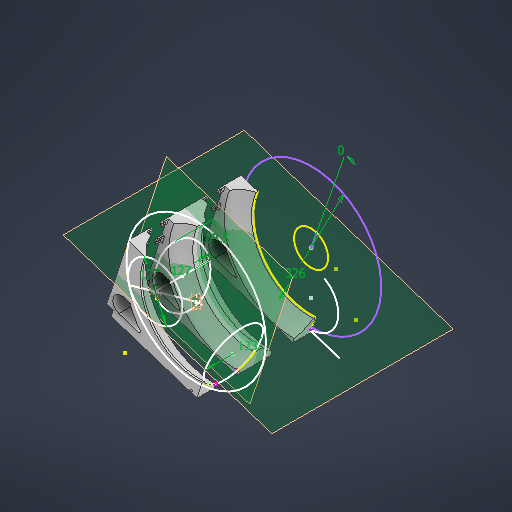
# Autodesk Inventor part: загиб 20-25
Saved by Autodesk Inventor 2025 (Build 290162000, 162)
## iProperties
Created: 2025-10-03
Part Number: загиб 20-25
Material: Типовые
Document SubType Name: Modeling
Designer: Phantom
Density: 1 g/cm^3
Appearance: По умолчанию
Author: Phantom
Autodesk Inventor part; units mm, degrees
ref_plane "YZ Plane" through (0, 0, 0) normal (1, 0, 0) x (0, 1, 0)
ref_plane "XZ Plane" through (0, 0, 0) normal (0, 1, 0) x (-1, 0, 0)
ref_plane "XY Plane" through (0, 0, 0) normal (0, 0, 1) x (1, 0, 0)
sketch "Эскиз1" plane through (0, 0, 0) normal (0, 0, 1) x (1, 0, 0)
  line L0 (14.5513, 220.3235) -> (16.6686, 220.3036)
  line L1 (220, 0) -> (230, 0) construction
  line L2 (0, 0) -> (170, 0)
  line L3 (170, 0) -> (170, 2)
  arc A0 (14.5513, 220.3235) -> (170, 0) centre (170, 165) ccw
  arc A1 (16.6686, 220.3036) -> (170, 2) centre (170, 165) ccw
  line L4 (170, 1) -> (170, 0)
  dimension "d12" = 330
  dimension "d13" = 2
  constraints: 10 end point, 4 point on circle, 2 centre point, 2 horizontal, 1 midpoint, 1 vertical
  measures "d12" diameter of A0
  measures "d13" radial gap between concentric circles of A0 A1
extrude "Выдавливание1" add sketch "Эскиз1" along normal blind 385
sketch "Эскиз2" plane through (0, 0, 0) normal (0, 0, -1) x (-1, 0, 0)
  line L0 (-16.6686, 220.3036) -> (-14.5513, 220.3235) projected
  arc A0 (-170, 2) -> (-16.6686, 220.3036) centre (-170, 165) ccw projected
  line L1 (-170, 0) -> (-170, 2) projected
  arc A1 (-170, 0) -> (-14.5513, 220.3235) centre (-170, 165) ccw projected
  point P0 (0, 0)
extrude "Выдавливание2" cut sketch "Эскиз2" against normal blind 121
chamfer "Фаска1" distance 2 angle 45 1 edges at (170, 2, 253)
chamfer "Фаска2" distance 2.8 angle 45 1 edges at (168.0001, 2.0123, 253)
sketch "Эскиз4" plane through (0, 0, 385) normal (0, 0, 1) x (1, 0, 0)
  line L0 (165.2006, 2.0707) -> (169.9739, 0.0263) projected
  arc A0 (16.6686, 220.3036) -> (165.2006, 2.0707) centre (170, 165) ccw projected
  line L1 (16.6686, 220.3036) -> (14.5513, 220.3235) projected
  arc A1 (14.5513, 220.3235) -> (170, 0) centre (170, 165) ccw projected
  line L2 (169.9739, 0.0263) -> (170, 0) projected
  arc A2 (8.48, 230.7703) -> (172.1929, 23.6823) centre (165.364, 186.5392) ccw projected
  arc A3 (6.3666, 230.6392) -> (177.1276, 21.959) centre (165.364, 186.5392) ccw projected
  line L3 (8.48, 230.7703) -> (6.3666, 230.6392) projected
  point P0 (0, 0)
  point P1 (6.736, 141.1283)
  point P2 (5.2437, 156.0352)
extrude "Выдавливание3" add sketch "Эскиз4" against normal up to surface (264 mm away) contours A3 L3 A2 A1
sketch "Эскиз5" plane through (0, 0, 385) normal (0, 0, 1) x (1, 0, 0)
  point P0 (0, 0)
sketch "Эскиз6" plane through (0, 0, 385) normal (0, 0, 1) x (1, 0, 0)
  arc A0 (8.48, 230.7703) -> (172.1929, 23.6823) centre (165.364, 186.5392) ccw projected
  arc A1 (4.2174, 151.0884) -> (177.1276, 21.959) centre (165.364, 186.5392) ccw projected
  arc A2 (6.3666, 230.6392) -> (6.736, 141.1283) centre (165.364, 186.5392) ccw projected
  line L0 (8.48, 230.7703) -> (6.3666, 230.6392) projected
  line L1 (165.2006, 2.0707) -> (169.9739, 0.0263) projected
  arc A3 (16.6686, 220.3036) -> (165.2006, 2.0707) centre (170, 165) ccw projected
  line L2 (16.6686, 220.3036) -> (14.5513, 220.3235) projected
  arc A4 (14.5513, 220.3235) -> (5.2437, 156.0352) centre (170, 165) ccw projected
  arc A5 (8.48, 230.7703) -> (5.2437, 156.0352) centre (165.364, 186.5392) ccw projected
  line L3 (8.48, 230.7703) -> (6.3666, 230.6392) projected
  arc A6 (6.3666, 230.6392) -> (6.736, 141.1283) centre (165.364, 186.5392) ccw projected
  arc A7 (6.736, 141.1283) -> (170, 0) centre (170, 165) ccw projected
  line L4 (169.9739, 0.0263) -> (170, 0) projected
  point P0 (0, 0)
  point P1 (5.2437, 156.0352)
  point P2 (8.6956, 141.5501)
extrude "Выдавливание4" cut sketch "Эскиз6" against normal through all contours A4 L2 A3 A0
sketch "Эскиз7" plane through (0, 0, 385) normal (0, 0, 1) x (1, 0, 0)
  arc A0 (8.48, 230.7703) -> (8.6956, 141.5501) centre (165.364, 186.5392) ccw projected
  line L0 (8.48, 230.7703) -> (6.3666, 230.6392) projected
  arc A1 (6.3666, 230.6392) -> (6.736, 141.1283) centre (165.364, 186.5392) ccw projected
  arc A2 (6.736, 141.1283) -> (170, 0) centre (170, 165) ccw projected
  line L1 (169.9739, 0.0263) -> (170, 0) projected
  line L2 (165.2006, 2.0707) -> (169.9739, 0.0263) projected
  arc A3 (8.6956, 141.5501) -> (165.2006, 2.0707) centre (170, 165) ccw projected
  line L3 (7.9507, 133.9351) -> (-40.0993, 149.5316)
  line L4 (-49.858, 62.7801) -> (67.4599, 424.2168) projected
  line L5 (-49.858, 62.7801) -> (127.0544, 5.6869)
  line L6 (-49.858, 62.7801) -> (-48.0056, 68.487)
  line L7 (-48.0056, 68.487) -> (101.3216, 20.2961)
  line L8 (86.2538, 25.1587) -> (84.4111, 19.4487)
  line L9 (-13.7205, 69.3639) -> (64.1078, 44.2472)
  line L10 (-13.7205, 69.3639) -> (-53.2073, 82.1071)
  line L11 (6.3666, 230.6392) -> (-61.8212, 20.5641)
  line L12 (0.3654, 112.7603) -> (33.0364, 102.1557)
  line L13 (0.3654, 112.7603) -> (-39.1966, 125.6017)
  point P0 (0, 0)
  point P1 (-42.9225, 78.788)
  point P2 (-48.2834, 62.2719)
  point P3 (85.6236, 23.2057)
  point P4 (54.2251, 47.4365)
  point P5 (-21.8795, 143.6177)
  point P6 (-28.8205, 122.2337)
  point P7 (15.1754, 107.9532)
  dimension "d24" = 6
  constraints: 20 end point, 4 parallel, 3 point on circle, 3 point on line, 2 perpendicular, 1 collinear, 2 other
  measures "d24" distance of L4.start L6.end
extrude "Выдавливание5" add sketch "Эскиз7" against normal up to surface (264 mm away) contours A1 A2 L3 L11 | L3 A2 L12 L13 L11 | A2 L7 L11 L10 L9 | A2 L8 L5 L11 L7
sketch "Эскиз8" plane through (0, 0, 385) normal (0, 0, 1) x (1, 0, 0)
  arc A0 (-12.5279, 69.512) -> (1.2437, 111.9401) centre (-8.4636, 91.6419) ccw projected
  arc A1 (15.1754, 107.9532) -> (54.2251, 47.4365) centre (170, 165) ccw projected
  arc A2 (9.1771, 109.9002) -> (50.7168, 43.874) centre (170, 165) ccw
  line L0 (-28.8205, 122.2337) -> (15.1754, 107.9532) projected
  line L1 (54.2251, 47.4365) -> (-42.9225, 78.788) projected
  point P0 (0, 0)
  point P1 (44.1807, 50.678)
  dimension "d27" = 5
  constraints: 2 point on circle, 1 centre point, 1 point on line
  measures "d27" radial gap between concentric circles of A1 A2
extrude "Выдавливание6" add sketch "Эскиз8" against normal up to surface (264 mm away)
sketch "Эскиз9" plane through (0, 0, 385) normal (0, 0, 1) x (1, 0, 0)
  arc A0 (8.48, 230.7703) -> (8.6956, 141.5501) centre (165.364, 186.5392) ccw projected
  line L0 (8.48, 230.7703) -> (6.3666, 230.6392) projected
  line L1 (6.3666, 230.6392) -> (-28.8205, 122.2337) projected
  line L2 (-28.8205, 122.2337) -> (9.1771, 109.9002) projected
  arc A1 (9.1771, 109.9002) -> (44.1807, 50.678) centre (170, 165) ccw projected
  line L3 (44.1807, 50.678) -> (-42.9225, 78.788) projected
  line L4 (-42.9225, 78.788) -> (-48.2834, 62.2719) projected
  line L5 (-48.2834, 62.2719) -> (84.4111, 19.4487) projected
  line L6 (84.4111, 19.4487) -> (85.6236, 23.2057) projected
  arc A2 (85.6236, 23.2057) -> (170, 0) centre (170, 165) ccw projected
  line L7 (169.9739, 0.0263) -> (170, 0) projected
  line L8 (165.2006, 2.0707) -> (169.9739, 0.0263) projected
  arc A3 (8.6956, 141.5501) -> (165.2006, 2.0707) centre (170, 165) ccw projected
  line L9 (85.6236, 23.2057) -> (90.4504, 38.1623)
  line L10 (84.4111, 19.4487) -> (85.6236, 23.2057) projected
  point P0 (0, 0)
  point P1 (86.2538, 25.1587)
  constraints: 2 end point, 1 collinear
extrude "Выдавливание7" cut sketch "Эскиз9" against normal through all contours A3 L8 L7 A2 L9
sketch "Эскиз10" plane through (0, 0, 385) normal (0, 0, 1) x (1, 0, 0)
  line L0 (8.48, 230.7703) -> (6.3666, 230.6392) projected
  line L1 (-48.2834, 62.2719) -> (6.3666, 230.6392)
  line L2 (-48.2834, 62.2719) -> (96.336, 15.3303)
  line L3 (84.4111, 19.4487) -> (86.2538, 25.1587) projected
  arc A0 (8.6956, 141.5501) -> (86.2538, 25.1587) centre (170, 165) ccw projected
  arc A1 (8.48, 230.7703) -> (8.6956, 141.5501) centre (165.364, 186.5392) ccw projected
  line L4 (8.48, 230.7703) -> (6.3666, 230.6392) projected
  line L5 (6.3666, 230.6392) -> (-28.8205, 122.2337) projected
  line L6 (-28.8205, 122.2337) -> (9.1771, 109.9002) projected
  arc A2 (9.1771, 109.9002) -> (44.1807, 50.678) centre (170, 165) ccw projected
  line L7 (44.1807, 50.678) -> (-42.9225, 78.788) projected
  line L8 (-42.9225, 78.788) -> (-48.2834, 62.2719) projected
  line L9 (-48.2834, 62.2719) -> (84.4111, 19.4487) projected
  line L10 (84.4111, 19.4487) -> (83.7893, 17.522)
  line L11 (84.4111, 19.4487) -> (86.2538, 25.1587) projected
  point P0 (0, 0)
  point P1 (84.3387, 19.2244)
  constraints: 6 end point, 1 collinear, 1 perpendicular
extrude "Выдавливание8" add sketch "Эскиз10" against normal up to surface (264 mm away) contours L10 L2 L9
sketch "Эскиз13" plane through (0, 0, 121) normal (0, 0, -1) x (-1, 0, 0)
  arc A0 (18.116, 75.0583) -> (12.6723, 73.0313) centre (8.93, 91.404) ccw projected
  arc A1 (15.1818, 72.1432) -> (12.9717, 71.5614) centre (8.93, 91.404) ccw
  line L0 (8.93, 91.404) -> (31.1796, 22.8568)
  line L1 (42.9225, 78.788) -> (48.2834, 62.2719) projected
  line L2 (8.93, 91.404) -> (-2.0706, 125.2951)
  line L3 (28.8205, 122.2337) -> (-9.1771, 109.9002) projected
  line L4 (-44.1807, 50.678) -> (42.9225, 78.788) projected
  line L5 (-6.3666, 230.6392) -> (28.8205, 122.2337) projected
  line L6 (28.8205, 122.2337) -> (42.9225, 78.788)
  line L7 (-27.6965, 100.8055) -> (34.3413, 120.9422)
  line L8 (-44.935, 52.7423) -> (51.7275, 83.9372)
  arc A2 (-44.1807, 50.678) -> (-9.1771, 109.9002) centre (-170, 165) ccw projected
  point P0 (0, 0)
  point P1 (1.7728, 113.4543)
  point P2 (2.6782, 110.6648)
  point P3 (15.8599, 70.0544)
  point P4 (-10.4135, 106.4154)
  point P5 (2.6782, 110.6648)
  point P6 (-41.3188, 53.9093)
  point P7 (15.1818, 72.1432)
  dimension "d40" = 1.5
  constraints: 10 end point, 3 parallel, 2 point on circle, 2 tangent, 1 centre point, 1 point on line
  measures "d40" radial gap between concentric circles of A0 A1
ref_plane "РабПлоскость1" through (-48.2834, -7.7133, 385) normal (0, 0, -1) x (0.3087313, 0.9511493, 0)
extrude "Выдавливание11" add sketch "Эскиз13" against normal up to surface (264 mm away) contours L8 L6 L4 L0 | L0 L4 A2 L8 | A1 L7 L6 L8 | L7 A2 L3 L2 | L2 L3 L6 L7
fillet "Сопряжение1" radius 3 2 edges at (41.3188, 53.9093, 253) (10.4135, 106.4154, 253)
sketch "Эскиз14" plane through (0, 0, 385) normal (0, 0, 1) x (1, 0, 0)
  line L0 (8.48, 230.7703) -> (6.3666, 230.6392) projected
  line L1 (6.3666, 230.6392) -> (55.6278, 214.6497)
  line L2 (-48.2834, 62.2719) -> (84.3387, 19.2244) projected
  arc A0 (8.48, 230.7703) -> (8.6956, 141.5501) centre (165.364, 186.5392) ccw projected
  point P0 (0, 0)
  point P1 (8.2707, 230.0212)
  constraints: 2 end point, 1 parallel
extrude "Выдавливание12" cut sketch "Эскиз14" against normal through all
sketch "Эскиз15" plane through (6.3666, 230.6392, 385) normal (0.3087313, 0.9511493, 0) x (0.9511493, -0.3087313, 0)
  line L0 (139.423, 0) -> (29.7199, 0) projected
  line L1 (139.423, 264) -> (29.7199, 264) projected
  line L2 (77.6819, 264) -> (77.6819, 0) projected
  line L3 (28.4369, 264) -> (28.4369, 0) projected
  line L4 (0, 264) -> (139.4335, 264) projected
  line L5 (139.4335, 0) -> (139.4335, 264) projected
  line L6 (0, 0) -> (139.4335, 0) projected
  line L7 (0, 0) -> (0, 264) projected
  line L8 (0, 0) -> (0, 40)
  line L9 (0, 40) -> (139.4335, 40)
  line L10 (0, 264) -> (0, 224)
  line L11 (0, 224) -> (139.4335, 224)
  line L12 (0, 132) -> (139.4335, 132)
  line L13 (0, 92) -> (139.4335, 92)
  line L14 (0, 172) -> (139.4335, 172)
  line L15 (28.4369, 264) -> (28.4369, 0) projected
  line L16 (28.4369, 92) -> (-4.7788, 92)
  line L17 (28.4369, 132) -> (-6.4168, 132)
  line L18 (28.4369, 172) -> (-6.4168, 172)
  point P0 (65.15, 385)
  point P1 (28.4369, 172)
  point P2 (139.4335, 172)
  point P3 (28.4369, 224)
  point P4 (28.4369, 92)
  point P5 (28.4369, 40)
  point P6 (139.4335, 92)
  point P7 (28.4369, 172)
  point P8 (28.4369, 92)
  dimension "d47" = 40
  dimension "d48" = 40
  dimension "d49" = 40
  dimension "d50" = 40
  constraints: 20 end point, 10 point on line, 3 midpoint, 2 parallel, 2 perpendicular, 1 horizontal
  measures "d47" distance of L6.start L8.end
  measures "d48" distance of L4.start L10.end
  measures "d49" distance between parallel lines of L12 L13
  measures "d50" distance between parallel lines of L12 L14
extrude "Выдавливание13" cut sketch "Эскиз15" against normal through all contours L9 L3 L13 L2 | L2 L13 L5 L9 | L9 L7 L13 L3 | L14 L3 L11 L2 | L2 L11 L5 L14 | L14 L7 L11 L3
sketch "Эскиз16" plane through (0, 0, 121) normal (0, 0, -1) x (-1, 0, 0)
  line L0 (-6.3666, 230.6392) -> (-8.2707, 230.0212) projected
  arc A0 (-8.6956, 141.5501) -> (-8.2707, 230.0212) centre (-165.364, 186.5392) ccw projected
  arc A1 (-86.2538, 25.1587) -> (-8.6956, 141.5501) centre (-170, 165) ccw projected
  line L1 (-86.2538, 25.1587) -> (-84.3387, 19.2244) projected
  line L2 (48.2834, 62.2719) -> (-84.3387, 19.2244) projected
  line L3 (-6.3666, 230.6392) -> (48.2834, 62.2719) projected
  arc A2 (-9.0336, 106.8633) -> (-10.9148, 105.0674) centre (-8.1075, 104.0098) ccw projected
  line L4 (-9.0336, 106.8633) -> (2.6782, 110.6648) projected
  arc A3 (15.1818, 72.1432) -> (2.6782, 110.6648) centre (8.93, 91.404) ccw projected
  line L5 (15.1818, 72.1432) -> (15.1818, 72.1432) projected
  line L6 (15.1818, 72.1432) -> (-31.6832, 57.0189) projected
  arc A4 (-34.9871, 61.6969) -> (-31.6832, 57.0189) centre (-32.6046, 59.8739) ccw projected
  arc A5 (-34.9871, 61.6969) -> (-10.9148, 105.0674) centre (-170, 165) ccw projected
  line L7 (-167.3298, -7.7134) -> (-261.1287, 281.2651)
  line L8 (-6.3666, 230.6392) -> (-234.3444, 156.6405)
  line L9 (-84.3387, 19.2244) -> (-167.3298, -7.7134)
  point P0 (0, 0)
  point P1 (-221.9798, 160.6539)
  dimension "d73" = 226.687
  constraints: 6 end point, 2 parallel
  measures "d73" distance between parallel lines of L3 L7
extrude "Выдавливание14" add sketch "Эскиз16" against normal up to surface (264 mm away) contours A0 A1 L1 L9 L7 L8
sketch "Эскиз17" plane through (0, 0, 385) normal (0, 0, 1) x (1, 0, 0)
  arc A0 (8.2707, 230.0212) -> (8.6956, 141.5501) centre (165.364, 186.5392) ccw projected
  line L0 (165.364, 186.5392) -> (8.6956, 141.5501)
  point P0 (0, 0)
  constraints: 2 end point, 1 coincident
ref_plane "РабПлоскость2" through (165.364, 186.5392, 385) normal (-0.9611557, -0.2760066, 0) x (0.2760066, -0.9611557, 0)
ref_plane "РабПлоскость3" through (165.364, 186.5392, 385) normal (0, 0, 1) x (1, 0, 0)
sketch "Эскиз18" plane through (165.364, 186.5392, 385) normal (0, 0, 1) x (1, 0, 0)
  circle A0 centre (0, 0) radius 163
  line L0 (0, 0) -> (-156.6684, -44.9891) projected
  circle A1 centre (-95.635, -27.4627) radius 63.5
  point P0 (-165.364, -186.5392)
  dimension "d55" = 127
  constraints: 1 centre point, 1 coincident, 1 point on line, 3 other
  measures "d55" diameter of A1
ref_plane "РабПлоскость4" through (69.729, 159.0765, 385) normal (-0.9611557, -0.2760066, 0) x (0.2760066, -0.9611557, 0)
sketch "Эскиз19" plane through (69.729, 159.0765, 385) normal (-0.9611557, -0.2760066, 0) x (0.2760066, -0.9611557, 0)
  line L0 (0, 0) -> (0, -127)
  line L1 (0, -40) -> (0, 0) projected
  ellipse E0 centre (0, -63.5) end of major axis (0, 0) minor radius 63.5
  point P0 (133.6516, -385)
  dimension "d57" = 63.5
  dimension "d56" = 127
  constraints: 2 end point, 2 vertical, 1 midpoint, 1 vertical alignment, 2 other
  measures "d56" distance of L0.start L0.end
ref_plane "РабПлоскость6" through (8.6956, 141.5501, 121) normal (-0.3087313, -0.9511493, 0) x (0.9511493, -0.3087313, 0)
sketch "Эскиз20" plane through (8.6956, 141.5501, 121) normal (-0.3087313, -0.9511493, 0) x (0.9511493, -0.3087313, 0)
  circle A0 centre (62.6409, 200.5) radius 66.5
  line L0 (196.9671, 0) -> (196.9671, 264) projected
  line L1 (196.9671, 132) -> (-88.0095, 132)
  circle A1 centre (62.6409, 63.5) radius 66.5
  line L2 (87.6409, 200.5) -> (87.6409, 175.2953)
  point P0 (35.4301, -121)
  dimension "d58" = 133
  dimension "d72" = 25
  constraints: 4 end point, 2 centre point, 1 coincident, 1 horizontal, 1 midpoint, 1 symmetric about line, 1 vertical, 1 other
  measures "d58" diameter of A0
  measures "d72" distance of A0.centre L2.start
sketch "Эскиз21" plane through (0, 0, 121) normal (0, 0, -1) x (-1, 0, 0)
  arc A0 (-86.2538, 25.1587) -> (-8.6956, 141.5501) centre (-170, 165) ccw projected
  circle A1 centre (-170, 165) radius 163
  point P0 (0, 0)
  constraints: 1 centre point, 1 coincident, 1 concentric
sweep "Сдвиг1" cut profiles "Эскиз20" path "Эскиз21" path curves A1
sketch "Эскиз22" plane through (0, 0, 385) normal (0, 0, 1) x (1, 0, 0)
  arc A0 (69.3261, 210.2034) -> (188.0526, 56.13) centre (170, 165) ccw projected
  line L0 (182.711, 39.6735) -> (167.3298, -7.7134) projected
  line L1 (221.9798, 160.6539) -> (82.8103, 205.8266) projected
  line L2 (54.3995, 215.0483) -> (6.3666, 230.6392) projected
  line L3 (6.3666, 230.6392) -> (-48.2834, 62.2719) projected
  line L4 (-48.2834, 62.2719) -> (167.3298, -7.7134) projected
  line L5 (221.9798, 160.6539) -> (193.0496, 71.525) projected
  spline S0 degree 8 poles (80.89, 128.5546) (82.865, 123.7256) (85.1392, 119.0186) (87.7037, 114.4558) (90.5476, 110.0578) (93.6585, 105.8445) (97.0223, 101.8344) (100.6234, 98.045) (110.2581, 89.087) (116.5832, 84.2276) (123.357, 79.9736) (130.5112, 76.3722) (137.973, 73.4614) (145.6657, 71.2696) (153.5085, 69.8164) (165.3316, 68.758) (169.2643, 68.5902) (173.2033, 68.606) (177.1388, 68.8058) (181.0606, 69.1891) (184.9588, 69.7549) (188.8236, 70.5014) (192.6958, 71.4384) (192.7464, 71.4507) (192.7969, 71.463) (192.8475, 71.4754) (192.898, 71.4877) (192.9486, 71.5001) (192.9991, 71.5125) (193.0496, 71.525) knots 0 0 0 0 0 0 0 0 0 0.304396 0.304396 0.304396 0.304396 0.304396 0.304396 0.304396 0.767561 0.767561 0.767561 0.767561 0.767561 0.767561 0.767561 0.996964 0.996964 0.996964 0.996964 0.996964 0.996964 0.996964 1 1 1 1 1 1 1 1 1 projected
  spline S1 degree 8 poles (82.8103, 205.8266) (81.512, 203.0541) (80.3146, 200.2344) (79.2198, 197.3717) (78.2296, 194.4705) (77.3455, 191.5352) (76.5688, 188.5703) (75.9007, 185.5805) (74.0863, 175.8059) (73.3829, 168.9372) (73.2422, 162.0192) (73.6676, 155.1058) (74.6565, 148.2502) (76.2004, 141.5052) (78.2854, 134.9229) (80.89, 128.5546) knots 0 0 0 0 0 0 0 0 0 0.30792 0.30792 0.30792 0.30792 0.30792 0.30792 0.30792 1 1 1 1 1 1 1 1 1 projected
  line L6 (193.0496, 71.525) -> (188.0526, 56.13)
  line L7 (69.3261, 210.2034) -> (82.8103, 205.8266)
  point P0 (0, 0)
  point P1 (188.0526, 56.13)
  point P2 (69.3261, 210.2034)
  constraints: 4 end point, 1 perpendicular, 4 other
extrude "Выдавливание15" cut sketch "Эскиз22" against normal through all
sketch "Эскиз23" plane through (167.3298, -7.7134, 293) normal (0.9511493, -0.3087313, 0) x (0, 0, -1)
  line L0 (-92, 0) -> (-52, 0) projected
  line L1 (-92, 0) -> (-52, 0)
  line L2 (172, 177.0146) -> (172, 0) projected
  line L3 (172, 0) -> (132, 0)
  line L4 (132, 0) -> (132, 198.8982)
  line L5 (132, 198.8982) -> (172, 198.8982)
  line L6 (172, 198.8982) -> (172, 0)
  line L7 (-92, 0) -> (-52, 0)
  line L8 (-52, 0) -> (-52, 229.2687)
  line L9 (-52, 229.2687) -> (-92, 229.2687)
  line L10 (-92, 229.2687) -> (-92, 0)
  line L11 (0, 0) -> (80, 0) projected
  line L12 (40, 0) -> (0, 0)
  line L13 (0, 0) -> (0, 235.4738)
  line L14 (0, 235.4738) -> (40, 235.4738)
  line L15 (40, 235.4738) -> (40, 0)
  line L16 (40, 0) -> (80, 0)
  line L17 (80, 0) -> (80, 261.9984)
  line L18 (80, 261.9984) -> (40, 261.9984)
  line L19 (40, 261.9984) -> (40, 0)
  line L20 (172, 198.8982) -> (-211.179, 198.8982)
  line L21 (172, 0) -> (-92, 0)
  point P0 (293, -44.3233)
  point P1 (172, 49.8207)
  point P2 (0, 198.8982)
  point P3 (-52, 198.8982)
  point P4 (132, 198.8982)
  point P5 (80, 198.8982)
  dimension "d63" = 40
  dimension "d64" = 40
  dimension "d65" = 40
  constraints: 38 end point, 9 equal length, 6 horizontal, 4 perpendicular, 1 midpoint
  measures "d63" distance of L4.end L5.end
  measures "d64" distance of L9.end L8.end
  measures "d65" distance of L13.end L14.end
extrude "Выдавливание16" cut sketch "Эскиз23" against normal through all contours L8 L20 L13 L21 | L17 L20 L4 L21
sketch "Эскиз24" plane through (0, 0, 385) normal (0, 0, 1) x (1, 0, 0)
  arc A0 (69.3261, 210.2034) -> (188.0526, 56.13) centre (170, 165) ccw projected
  circle A1 centre (170, 165) radius 135
  point P0 (0, 0)
  point P1 (182.711, 39.6735)
  point P2 (54.3995, 215.0483)
  dimension "d68" = 270
  constraints: 1 centre point, 1 coincident
  measures "d68" diameter of A1
extrude "Выдавливание17" cut sketch "Эскиз24" against normal through all
sketch "Эскиз26" plane through (-48.2834, 62.2719, 213) normal (-0.9511493, 0.3087313, 0) x (0, 0, 1)
  line L0 (-52, 177.0146) -> (-52, 2.4876) projected
  line L1 (-52, 0) -> (-52, 177.0146) projected
  line L2 (0, 177.0146) -> (0, 0) projected
  line L3 (-52, 0) -> (-52, 50)
  circle A0 centre (-44, 50) radius 2.1
  line L4 (-37, 48) -> (-37, 52)
  line L5 (-41, 44) -> (-52, 44)
  line L6 (-41, 56) -> (-52, 56)
  arc A1 (-41, 44) -> (-37, 48) centre (-41, 48) ccw
  arc A2 (-37, 52) -> (-41, 56) centre (-41, 52) ccw
  line L7 (-52, 177.0146) -> (-52, 127.0146)
  circle A3 centre (-44, 127.0146) radius 2.1
  line L8 (-37, 125.0146) -> (-37, 129.0146)
  line L9 (-41, 121.0146) -> (-52, 121.0146)
  line L10 (-41, 133.0146) -> (-52, 133.0146)
  arc A4 (-41, 121.0146) -> (-37, 125.0146) centre (-41, 125.0146) ccw
  arc A5 (-37, 129.0146) -> (-41, 133.0146) centre (-41, 129.0146) ccw
  line L11 (80, 0) -> (0, 0) projected
  line L12 (40, 0) -> (40, 23)
  line L13 (121, 121.0146) -> (132, 121.0146)
  circle A6 centre (124, 127.0146) radius 2.1
  line L14 (121, 133.0146) -> (132, 133.0146)
  arc A7 (117, 125.0146) -> (121, 121.0146) centre (121, 125.0146) ccw
  line L15 (117, 125.0146) -> (117, 129.0146)
  arc A8 (121, 133.0146) -> (117, 129.0146) centre (121, 129.0146) ccw
  line L16 (132, 177.0146) -> (132, 0) projected
  line L17 (162.0468, 235) -> (162.0468, 380) projected
  line L18 (235.0468, 380) -> (162.0468, 380) projected
  line L19 (235.0468, 0) -> (235.0468, 380) projected
  line L20 (52.056, 0) -> (235.0468, 0) projected
  line L21 (52.056, 0) -> (52.056, 25.8521) projected
  line L22 (52.056, 25.8521) -> (-62.9532, 25.8521) projected
  line L23 (-62.9532, 25.8521) -> (-62.9532, 0) projected
  line L24 (-154.9532, 0) -> (-62.9532, 0) projected
  line L25 (-154.9532, 380) -> (-154.9532, 0) projected
  line L26 (-81.9532, 380) -> (-154.9532, 380) projected
  line L27 (-81.9532, 380) -> (-81.9532, 235) projected
  line L28 (-81.9532, 235) -> (162.0468, 235) projected
  arc A9 (181.5468, 115.5763) -> (183.5468, 113.5763) centre (183.5468, 115.5763) ccw projected
  line L29 (183.5468, 113.5763) -> (212.1996, 113.5763) projected
  arc A10 (212.1996, 113.5763) -> (213.8265, 116.7395) centre (212.1996, 115.5763) ccw projected
  line L30 (213.8265, 116.7395) -> (185.1737, 156.8147) projected
  arc A11 (185.1737, 156.8147) -> (181.5468, 155.6515) centre (183.5468, 155.6515) ccw projected
  line L31 (181.5468, 155.6515) -> (181.5468, 115.5763) projected
  arc A12 (181.5468, 288.4236) -> (183.5468, 286.4236) centre (183.5468, 288.4236) ccw projected
  line L32 (183.5468, 286.4236) -> (212.1996, 286.4236) projected
  arc A13 (212.1996, 286.4236) -> (213.8265, 289.5868) centre (212.1996, 288.4236) ccw projected
  line L33 (213.8265, 289.5868) -> (185.1737, 329.662) projected
  arc A14 (185.1737, 329.662) -> (181.5468, 328.4988) centre (183.5468, 328.4988) ccw projected
  line L34 (181.5468, 328.4988) -> (181.5468, 288.4236) projected
  line L35 (-132.106, 113.5763) -> (-103.4532, 113.5763) projected
  arc A15 (-103.4532, 113.5763) -> (-101.4532, 115.5763) centre (-103.4532, 115.5763) ccw projected
  line L36 (-101.4532, 115.5763) -> (-101.4532, 155.6515) projected
  arc A16 (-101.4532, 155.6515) -> (-105.0802, 156.8147) centre (-103.4532, 155.6515) ccw projected
  line L37 (-105.0802, 156.8147) -> (-133.733, 116.7395) projected
  arc A17 (-133.733, 116.7395) -> (-132.106, 113.5763) centre (-132.106, 115.5763) ccw projected
  line L38 (-132.106, 286.4236) -> (-103.4532, 286.4236) projected
  arc A18 (-103.4532, 286.4236) -> (-101.4532, 288.4236) centre (-103.4532, 288.4236) ccw projected
  line L39 (-101.4532, 288.4236) -> (-101.4532, 328.4988) projected
  arc A19 (-101.4532, 328.4988) -> (-105.0802, 329.662) centre (-103.4532, 328.4988) ccw projected
  line L40 (-105.0802, 329.662) -> (-133.733, 289.5868) projected
  arc A20 (-133.733, 289.5868) -> (-132.106, 286.4236) centre (-132.106, 288.4236) ccw projected
  arc A21 (-138.4532, 209.6747) -> (-134.8263, 208.5115) centre (-136.4532, 209.6747) ccw projected
  line L41 (-134.8263, 208.5115) -> (-107.9144, 248.5867) projected
  arc A22 (-107.9144, 248.5867) -> (-109.5414, 251.7499) centre (-109.5414, 249.7499) ccw projected
  line L42 (-109.5414, 251.7499) -> (-136.4532, 251.7499) projected
  arc A23 (-136.4532, 251.7499) -> (-138.4532, 249.7499) centre (-136.4532, 249.7499) ccw projected
  line L43 (-138.4532, 249.7499) -> (-138.4532, 209.6747) projected
  arc A24 (-133.733, 19.2632) -> (-132.106, 16.1) centre (-132.106, 18.1) ccw projected
  line L44 (-132.106, 16.1) -> (-103.4532, 16.1) projected
  arc A25 (-103.4532, 16.1) -> (-101.4532, 18.1) centre (-103.4532, 18.1) ccw projected
  line L45 (-101.4532, 18.1) -> (-101.4532, 58.1752) projected
  arc A26 (-101.4532, 58.1752) -> (-105.0802, 59.3385) centre (-103.4532, 58.1752) ccw projected
  line L46 (-105.0802, 59.3385) -> (-133.733, 19.2632) projected
  arc A27 (218.5468, 249.7499) -> (216.5468, 251.7499) centre (216.5468, 249.7499) ccw projected
  line L47 (216.5468, 251.7499) -> (189.6349, 251.7499) projected
  arc A28 (189.6349, 251.7499) -> (188.008, 248.5867) centre (189.6349, 249.7499) ccw projected
  line L48 (188.008, 248.5867) -> (214.9198, 208.5115) projected
  arc A29 (214.9198, 208.5115) -> (218.5468, 209.6747) centre (216.5468, 209.6747) ccw projected
  line L49 (218.5468, 209.6747) -> (218.5468, 249.7499) projected
  line L50 (183.5468, 16.1) -> (212.1996, 16.1) projected
  arc A30 (212.1996, 16.1) -> (213.8265, 19.2632) centre (212.1996, 18.1) ccw projected
  line L51 (213.8265, 19.2632) -> (185.1737, 59.3385) projected
  arc A31 (185.1737, 59.3385) -> (181.5468, 58.1752) centre (183.5468, 58.1752) ccw projected
  line L52 (181.5468, 58.1752) -> (181.5468, 18.1) projected
  arc A32 (181.5468, 18.1) -> (183.5468, 16.1) centre (183.5468, 18.1) ccw projected
  arc A33 (214.9198, 122.0878) -> (218.5468, 123.251) centre (216.5468, 123.251) ccw projected
  line L53 (218.5468, 123.251) -> (218.5468, 163.3263) projected
  arc A34 (218.5468, 163.3263) -> (216.5468, 165.3263) centre (216.5468, 163.3263) ccw projected
  line L54 (216.5468, 165.3263) -> (189.6349, 165.3263) projected
  arc A35 (189.6349, 165.3263) -> (188.008, 162.1631) centre (189.6349, 163.3263) ccw projected
  line L55 (188.008, 162.1631) -> (214.9198, 122.0878) projected
  arc A36 (218.5468, 336.1736) -> (216.5468, 338.1736) centre (216.5468, 336.1736) ccw projected
  line L56 (216.5468, 338.1736) -> (189.6349, 338.1736) projected
  arc A37 (189.6349, 338.1736) -> (188.008, 335.0103) centre (189.6349, 336.1736) ccw projected
  line L57 (188.008, 335.0103) -> (214.9198, 294.9351) projected
  arc A38 (214.9198, 294.9351) -> (218.5468, 296.0983) centre (216.5468, 296.0983) ccw projected
  line L58 (218.5468, 296.0983) -> (218.5468, 336.1736) projected
  arc A39 (-138.4532, 123.251) -> (-134.8263, 122.0878) centre (-136.4532, 123.251) ccw projected
  line L59 (-134.8263, 122.0878) -> (-107.9144, 162.1631) projected
  arc A40 (-107.9144, 162.1631) -> (-109.5414, 165.3263) centre (-109.5414, 163.3263) ccw projected
  line L60 (-109.5414, 165.3263) -> (-136.4532, 165.3263) projected
  arc A41 (-136.4532, 165.3263) -> (-138.4532, 163.3263) centre (-136.4532, 163.3263) ccw projected
  line L61 (-138.4532, 163.3263) -> (-138.4532, 123.251) projected
  arc A42 (-138.4532, 296.0983) -> (-134.8263, 294.9351) centre (-136.4532, 296.0983) ccw projected
  line L62 (-134.8263, 294.9351) -> (-107.9144, 335.0103) projected
  arc A43 (-107.9144, 335.0103) -> (-109.5414, 338.1736) centre (-109.5414, 336.1736) ccw projected
  line L63 (-109.5414, 338.1736) -> (-136.4532, 338.1736) projected
  arc A44 (-136.4532, 338.1736) -> (-138.4532, 336.1736) centre (-136.4532, 336.1736) ccw projected
  line L64 (-138.4532, 336.1736) -> (-138.4532, 296.0983) projected
  line L65 (-132.106, 199.9999) -> (-103.4532, 199.9999) projected
  arc A45 (-103.4532, 199.9999) -> (-101.4532, 201.9999) centre (-103.4532, 201.9999) ccw projected
  line L66 (-101.4532, 201.9999) -> (-101.4532, 242.0752) projected
  arc A46 (-101.4532, 242.0752) -> (-105.0802, 243.2384) centre (-103.4532, 242.0752) ccw projected
  line L67 (-105.0802, 243.2384) -> (-133.733, 203.1631) projected
  arc A47 (-133.733, 203.1631) -> (-132.106, 199.9999) centre (-132.106, 201.9999) ccw projected
  arc A48 (-138.4532, 25.7748) -> (-134.8263, 24.6115) centre (-136.4532, 25.7748) ccw projected
  line L68 (-134.8263, 24.6115) -> (-107.9144, 64.6868) projected
  arc A49 (-107.9144, 64.6868) -> (-109.5414, 67.85) centre (-109.5414, 65.85) ccw projected
  line L69 (-109.5414, 67.85) -> (-136.4532, 67.85) projected
  arc A50 (-136.4532, 67.85) -> (-138.4532, 65.85) centre (-136.4532, 65.85) ccw projected
  line L70 (-138.4532, 65.85) -> (-138.4532, 25.7748) projected
  arc A51 (181.5468, 201.9999) -> (183.5468, 199.9999) centre (183.5468, 201.9999) ccw projected
  line L71 (183.5468, 199.9999) -> (212.1996, 199.9999) projected
  arc A52 (212.1996, 199.9999) -> (213.8265, 203.1631) centre (212.1996, 201.9999) ccw projected
  line L72 (213.8265, 203.1631) -> (185.1737, 243.2384) projected
  arc A53 (185.1737, 243.2384) -> (181.5468, 242.0752) centre (183.5468, 242.0752) ccw projected
  line L73 (181.5468, 242.0752) -> (181.5468, 201.9999) projected
  line L74 (216.5468, 67.85) -> (189.6349, 67.85) projected
  arc A54 (189.6349, 67.85) -> (188.008, 64.6868) centre (189.6349, 65.85) ccw projected
  line L75 (188.008, 64.6868) -> (214.9198, 24.6115) projected
  arc A55 (214.9198, 24.6115) -> (218.5468, 25.7748) centre (216.5468, 25.7748) ccw projected
  line L76 (218.5468, 25.7748) -> (218.5468, 65.85) projected
  arc A56 (218.5468, 65.85) -> (216.5468, 67.85) centre (216.5468, 65.85) ccw projected
  circle A57 centre (-92.4532, 373.8998) radius 1.625 projected
  circle A58 centre (-92.4532, 189.9999) radius 1.625 projected
  circle A59 centre (-92.4532, 6.1) radius 1.625 projected
  circle A60 centre (-147.4532, 103.5763) radius 1.625 projected
  circle A61 centre (-147.4532, 276.4236) radius 1.625 projected
  circle A62 centre (-147.4532, 189.9999) radius 1.625 projected
  circle A63 centre (-147.4532, 373.8998) radius 1.625 projected
  circle A64 centre (-147.4532, 6.1) radius 1.625 projected
  circle A65 centre (-92.4532, 103.5763) radius 1.625 projected
  circle A66 centre (-92.4532, 276.4236) radius 1.625 projected
  circle A67 centre (227.5468, 103.5763) radius 1.625 projected
  circle A68 centre (227.5468, 373.8998) radius 1.625 projected
  circle A69 centre (227.5468, 276.4236) radius 1.625 projected
  circle A70 centre (227.5468, 189.9999) radius 1.625 projected
  circle A71 centre (227.5468, 6.1) radius 1.625 projected
  circle A72 centre (172.5468, 189.9999) radius 1.625 projected
  circle A73 centre (172.5468, 103.5763) radius 1.625 projected
  circle A74 centre (172.5468, 373.8998) radius 1.625 projected
  circle A75 centre (172.5468, 6.1) radius 1.625 projected
  circle A76 centre (172.5468, 276.4236) radius 1.625 projected
  line L77 (-52, 0) -> (0, 0)
  line L78 (-26, 0) -> (-26, 11.5)
  circle A77 centre (-8, 50) radius 2.1
  line L79 (-15, 48) -> (-15, 52)
  line L80 (-11, 44) -> (0, 44)
  line L81 (-11, 56) -> (0, 56)
  arc A78 (-15, 48) -> (-11, 44) centre (-11, 48) ccw
  arc A79 (-11, 56) -> (-15, 52) centre (-11, 52) ccw
  line L82 (-11, 121.0146) -> (0, 121.0146)
  circle A80 centre (-8, 127.0146) radius 2.1
  line L83 (-11, 133.0146) -> (0, 133.0146)
  arc A81 (-15, 125.0146) -> (-11, 121.0146) centre (-11, 125.0146) ccw
  line L84 (-15, 125.0146) -> (-15, 129.0146)
  arc A82 (-11, 133.0146) -> (-15, 129.0146) centre (-11, 129.0146) ccw
  line L85 (91, 10) -> (80, 10)
  arc A83 (91, 10) -> (95, 14) centre (91, 14) ccw
  line L86 (95, 14) -> (95, 18)
  arc A84 (95, 18) -> (91, 22) centre (91, 18) ccw
  circle A85 centre (88, 16) radius 2.1
  line L87 (91, 22) -> (80, 22)
  line L88 (91, 121.0146) -> (80, 121.0146)
  circle A86 centre (88, 127.0146) radius 2.1
  line L89 (91, 133.0146) -> (80, 133.0146)
  arc A87 (91, 121.0146) -> (95, 125.0146) centre (91, 125.0146) ccw
  line L90 (95, 125.0146) -> (95, 129.0146)
  arc A88 (95, 129.0146) -> (91, 133.0146) centre (91, 129.0146) ccw
  line L91 (80, 0) -> (80, 177.0146) projected
  line L92 (172, 0) -> (132, 0) projected
  line L93 (80, 0) -> (132, 0)
  line L94 (106, 0) -> (106, 7.725)
  line L95 (121, 22) -> (132, 22)
  circle A89 centre (124, 16) radius 2.1
  line L96 (121, 10) -> (132, 10)
  arc A90 (121, 22) -> (117, 18) centre (121, 18) ccw
  line L97 (117, 14) -> (117, 18)
  arc A91 (117, 14) -> (121, 10) centre (121, 14) ccw
  line L98 (-41, 165.0146) -> (-52, 165.0146)
  circle A92 centre (-44, 171.0146) radius 2.1
  line L99 (-41, 177.0146) -> (-52, 177.0146)
  arc A93 (-41, 165.0146) -> (-37, 169.0146) centre (-41, 169.0146) ccw
  line L100 (-37, 169.0146) -> (-37, 173.0146)
  arc A94 (-37, 173.0146) -> (-41, 177.0146) centre (-41, 173.0146) ccw
  line L101 (-15, 169.0146) -> (-15, 173.0146)
  arc A95 (-15, 169.0146) -> (-11, 165.0146) centre (-11, 169.0146) ccw
  arc A96 (-11, 177.0146) -> (-15, 173.0146) centre (-11, 173.0146) ccw
  line L102 (-11, 177.0146) -> (0, 177.0146)
  line L103 (-11, 165.0146) -> (0, 165.0146)
  circle A97 centre (-8, 171.0146) radius 2.1
  line L104 (117, 169.0146) -> (117, 173.0146)
  arc A98 (117, 169.0146) -> (121, 165.0146) centre (121, 169.0146) ccw
  arc A99 (121, 177.0146) -> (117, 173.0146) centre (121, 173.0146) ccw
  line L105 (121, 177.0146) -> (132, 177.0146)
  line L106 (121, 165.0146) -> (132, 165.0146)
  circle A100 centre (124, 171.0146) radius 2.1
  line L107 (91, 177.0146) -> (80, 177.0146)
  arc A101 (95, 173.0146) -> (91, 177.0146) centre (91, 173.0146) ccw
  circle A102 centre (88, 171.0146) radius 2.1
  line L108 (95, 169.0146) -> (95, 173.0146)
  line L109 (91, 165.0146) -> (80, 165.0146)
  arc A103 (91, 165.0146) -> (95, 169.0146) centre (91, 169.0146) ccw
  point P0 (-213, -44.3233)
  point P1 (-52, 10.6203)
  point P2 (-52, 127.0146)
  point P3 (132, 44)
  point P4 (132, 56)
  point P5 (132, 127.0146)
  point P6 (132, 127.0146)
  point P7 (0, 50)
  point P8 (0, 127.0146)
  point P9 (0, 127.0146)
  point P10 (80, 50)
  point P11 (80, 127.0146)
  point P12 (80, 127.0146)
  point P13 (0, 121.0146)
  point P14 (0, 133.0146)
  point P15 (-52, 133.0146)
  point P16 (-52, 121.0146)
  point P17 (0, 56)
  point P18 (-52, 56)
  point P19 (85.5, 10)
  point P20 (126.5, 10)
  point P21 (132, 22)
  point P22 (-52, 171.0146)
  point P23 (-52, 171.0146)
  point P24 (0, 177.0146)
  point P25 (0, 171.0146)
  point P26 (0, 171.0146)
  point P27 (132, 177.0146)
  point P28 (132, 171.0146)
  point P29 (132, 171.0146)
  point P30 (80, 177.0146)
  point P31 (80, 171.0146)
  point P32 (80, 171.0146)
  point P33 (132, 165.0146)
  point P34 (80, 165.0146)
  point P35 (0, 165.0146)
  point P36 (-52, 177.0146)
  point P37 (-52, 165.0146)
  dimension "d77" = 4.2
  dimension "d78" = 15
  dimension "d80" = 4
  dimension "d81" = 50
  dimension "d82" = 4.2
  dimension "d83" = 4
  dimension "d88" = 10
  dimension "d89" = 6
  dimension "d115" = 4.2
  dimension "d116" = 4
  constraints: 92 symmetric about line, 86 end point, 48 point on circle, 36 centre point, 12 tangent, 7 horizontal, 6 vertical, 4 midpoint, 3 equal radius, 3 point on line, 1 collinear, 1 perpendicular, 25 other
  measures "d77" diameter of A0
  measures "d78" distance between parallel lines of L0 L4
  measures "d80" radius of A1
  measures "d81" distance of L0.start L7.end
  measures "d82" diameter of A3
  measures "d83" radius of A4
  measures "d88" distance between parallel lines of L20 L85
  measures "d89" vertical distance of point (85.5, 10) A85.centre
  measures "d115" diameter of A92
  measures "d116" radius of A93
extrude "Выдавливание19" add sketch "Эскиз26" against normal blind 3.2 contours L99 A94 L100 A93 L98 L0 | L10 A5 L8 A4 L9 L0 | L6 A2 L4 A1 L5 L0 | L2 L103 A95 L101 A96 L102 | L2 L82 A81 L84 A82 L83 | L2 L80 A78 L79 A79 L81 | A7 L15 A8 L14 L16 L13 | L16 L106 A98 L104 A99 L105 | L16 L96 A91 L97 A90 L95 | L85 L91 L87 A84 L86 A83 | L88 L91 L89 A88 L90 A87 | L91 L107 A101 L108 A103 L109
fillet "Сопряжение3" radius 3 24 edges at (-5.6958, 188.2947, 161) (-6.0263, 182.0938, 161) (-9.4005, 176.8809, 161) (-29.8031, 108.8415, 161) (-29.4726, 115.0423, 161) (-33.1774, 103.6285, 161) (-6.0263, 182.0938, 213) (-29.8031, 108.8415, 213) (-29.4726, 115.0423, 213) (-5.6958, 188.2947, 213) (-40.3, 76.5024, 345) (-6.0263, 182.0938, 345) (-5.6958, 188.2947, 345) (-9.4005, 176.8809, 345) (-6.0263, 182.0938, 293) (-40.3, 76.5024, 293) (-43.6742, 71.2895, 293) (-9.4005, 176.8809, 293) (-39.9694, 82.7032, 293) (-5.6958, 188.2947, 293) (-39.9694, 82.7032, 345) (-43.6742, 71.2895, 345) (-9.4005, 176.8809, 213) (-33.1774, 103.6285, 213)
sketch "Эскиз27" plane through (-48.2834, 62.2719, 345) normal (-0.3087313, -0.9511493, 0) x (0.9511493, -0.3087313, 0)
  line L0 (0, 0) -> (226.687, 0) projected
  line L1 (226.687, -224) -> (226.687, -184) projected
  line L2 (0, 40) -> (226.687, 40) projected
  line L3 (0, 40) -> (0, 0) projected
  line L4 (226.687, -184) -> (0, -184) projected
  line L5 (0, -184) -> (0, -224) projected
  line L6 (0, -224) -> (226.687, -224) projected
  line L7 (226.687, -224) -> (226.687, -184) projected
  line L8 (215, 40) -> (215, 36)
  line L9 (226.687, 36) -> (211.687, 36)
  line L10 (211.687, 36) -> (211.687, 28)
  line L11 (206.687, 28) -> (216.687, 28)
  line L12 (216.687, 28) -> (216.687, 36)
  line L13 (216.687, 36) -> (206.687, 36)
  line L14 (206.687, 36) -> (206.687, 28)
  line L15 (206.687, 28) -> (216.687, 36) construction
  line L16 (216.687, 28) -> (206.687, 36) construction
  line L17 (226.687, -101.4522) -> (226.687, -82.5478) projected
  line L18 (226.687, -92) -> (183, -92)
  line L19 (215, -224) -> (215, -220)
  line L20 (211.687, -220) -> (211.687, -212)
  line L21 (206.687, -212) -> (216.687, -212)
  line L22 (216.687, -212) -> (216.687, -220)
  line L23 (216.687, -220) -> (206.687, -220)
  line L24 (206.687, -220) -> (206.687, -212)
  line L25 (206.687, -212) -> (216.687, -220) construction
  line L26 (216.687, -212) -> (206.687, -220) construction
  line L27 (0, 0) -> (226.687, 0) projected
  line L28 (226.687, 0) -> (226.687, 40) projected
  line L29 (0, 40) -> (226.687, 40) projected
  line L30 (0, 40) -> (0, 0) projected
  line L31 (226.687, -52) -> (0, -52) projected
  line L32 (0, -52) -> (0, -132) projected
  line L33 (0, -132) -> (226.687, -132) projected
  line L34 (226.687, -132) -> (226.687, -52) projected
  line L35 (226.687, 0) -> (226.687, 40) projected
  line L36 (226.687, -52) -> (0, -52) projected
  line L37 (0, -52) -> (0, -132) projected
  line L38 (0, -132) -> (226.687, -132) projected
  line L39 (226.687, -132) -> (226.687, -52) projected
  line L40 (226.687, -184) -> (0, -184) projected
  line L41 (0, -184) -> (0, -224) projected
  line L42 (0, -224) -> (226.687, -224) projected
  point P0 (65.15, -345)
  point P1 (211.687, 32)
  point P2 (211.687, 36)
  point P3 (211.687, -216)
  dimension "d90" = 4
  dimension "d91" = 15
  dimension "d92" = 8
  dimension "d93" = 10
  constraints: 36 end point, 9 symmetric about line, 4 midpoint, 3 horizontal, 3 point on line, 2 parallel, 2 vertical, 1 perpendicular
  measures "d90" distance of L8.start L8.end
  measures "d91" distance of L9.start L9.end
  measures "d92" distance of L9.end L10.end
  measures "d93" distance of L13.end L12.end
extrude "Выдавливание20" cut sketch "Эскиз27" against normal blind 10.2 contours L12 L11 L10 L9 | L10 L11 L14 L13 | L23 L24 L21 L20 | L20 L21 L22 L23
sketch "Эскиз28" plane through (0, 0, 385) normal (0, 0, 1) x (1, 0, 0)
  line L0 (157.8183, -4.6261) -> (148.3068, -1.5388) projected
  line L1 (157.8183, -4.6261) -> (160.9674, 5.0756) projected
  line L2 (160.9674, 5.0756) -> (151.4559, 8.1629) projected
  line L3 (148.3068, -1.5388) -> (151.4559, 8.1629) projected
  circle A0 centre (154.6371, 1.7684) radius 2.1
  point P0 (0, 0)
  dimension "d96" = 4.2
  constraints: 1 centre point
  measures "d96" diameter of A0
extrude "Выдавливание21" cut sketch "Эскиз28" against normal up to surface (12 mm away) contours A0
ref_plane "РабПлоскость7" through (167.3298, -7.7134, 253) normal (0, 0, -1) x (-0.9511493, 0.3087313, 0)
mirror "Зеркальное отражение1" about plane through (167.3298, -7.7134, 253) normal (0, 0, -1) of "Выдавливание21"
sketch "Эскиз29" plane through (0, 0, 121) normal (0, 0, -1) x (-1, 0, 0)
  arc A0 (-179.684, 30.3478) -> (-45.7741, 217.8481) centre (-170, 165) ccw projected
  line L0 (-171.2274, 4.2945) -> (-179.684, 30.3478) projected
  line L1 (-179.684, 30.3478) -> (-170.6086, 2.3881) projected
  point P0 (0, 0)
sketch "Эскиз30" plane through (0, 0, 121) normal (0, 0, -1) x (-1, 0, 0)
  arc A0 (-202.3114, 118.5304) -> (-138.3087, 8.8369) centre (-170.2798, 63.7013) ccw
  line L0 (-235.6189, -24.2683) -> (-32.8332, 41.5534)
  line L1 (-179.684, 30.3478) -> (-167.3298, -7.7134) projected
  circle A1 centre (-170.9101, 168.107) radius 163
  circle A2 centre (-169.8502, 165.0516) radius 40 projected
  line L2 (-169.8502, 165.0516) -> (-182.9647, 202.8576)
  point P0 (0, 0)
  dimension "d100" = 326
  dimension "d102" = 0
  constraints: 4 end point, 2 centre point, 2 point on circle, 2 tangent, 1 equal length, 1 perpendicular, 4 other
  measures "d100" diameter of A1
  measures "d102" distance from line of A1.centre L2
sketch "Эскиз32" plane through (6.3666, 230.6392, 293) normal (0.3087313, 0.9511493, 0) x (0.9511493, -0.3087313, 0)
  line L0 (0, 0) -> (0, 80) projected
  line L1 (0, 40) -> (226.687, 40)
  line L2 (226.687, 172) -> (226.687, 132) projected
  line L3 (0, 38.75) -> (226.687, 38.75)
  line L4 (0, 41.25) -> (226.687, 41.25)
  line L5 (226.687, 49.4522) -> (226.687, 30.5478) projected
  point P0 (65.15, 293)
  point P1 (226.687, 80)
  point P2 (226.687, 0)
  point P3 (226.687, 41.25)
  point P4 (0, 41.25)
  point P5 (0, 38.75)
  point P6 (226.687, 38.75)
  dimension "d105" = 1.25
  dimension "d106" = 1.25
  constraints: 6 end point, 2 parallel, 1 midpoint, 1 point on line
  measures "d105" distance between parallel lines of L1 L3
  measures "d106" distance between parallel lines of L1 L4
extrude "Выдавливание23" [suppressed]
sketch "Эскиз33" plane through (-48.2834, 62.2719, 345) normal (-0.3087313, -0.9511493, 0) x (0.9511493, -0.3087313, 0)
  line L0 (41.4314, 40) -> (0, 40) projected
  line L1 (0, 40) -> (16, 40)
  line L2 (16, 40) -> (16, 24)
  line L3 (16, 24) -> (0, 24)
  line L4 (0, 24) -> (0, 40)
  line L5 (0, -224) -> (226.687, -224) projected
  line L6 (0, -224) -> (16, -224)
  line L7 (16, -224) -> (16, -208)
  line L8 (16, -208) -> (0, -208)
  line L9 (0, -208) -> (0, -224)
  point P0 (65.15, -345)
  point P1 (16, -224)
  dimension "d109" = 16
  dimension "d110" = 16
  dimension "d111" = 16
  dimension "d112" = 16
  constraints: 16 end point, 4 parallel, 2 horizontal, 2 perpendicular
  measures "d109" distance of L2.end L3.end
  measures "d110" distance of L1.end L2.end
  measures "d111" distance of L8.end L7.end
  measures "d112" distance of L7.end L6.end
extrude "Выдавливание24" cut sketch "Эскиз33" against normal blind 16
sketch "Эскиз34" plane through (167.3298, -7.7134, 385) normal (0.9511493, -0.3087313, 0) x (0, 0, -1)
  circle A0 centre (62.326, 73.2606) radius 66.5
  point P0 (385, -44.3233)
  dimension "d117" = 133
  constraints: 1 centre point, 3 other
  measures "d117" diameter of A0
